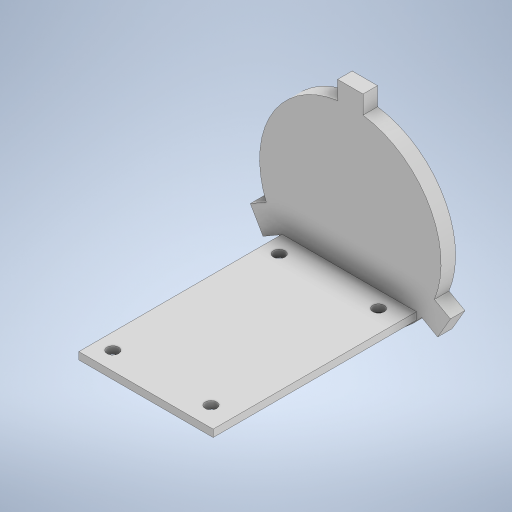
# Autodesk Inventor part: Electronic casing
Saved by Autodesk Inventor 2024 (Build 280153000, 153)
## iProperties
Created: 2024-03-27
Part Number: Electronic casing
Material: Generic
Document SubType Name: Modeling
Designer: auror
Density: 1 g/cm^3
Appearance: Default
Author: auror
Autodesk Inventor part; units mm, degrees
ref_plane "YZ Plane" through (0, 0, 0) normal (1, 0, 0) x (0, 1, 0)
ref_plane "XZ Plane" through (0, 0, 0) normal (0, 1, 0) x (-1, 0, 0)
ref_plane "XY Plane" through (0, 0, 0) normal (0, 0, 1) x (1, 0, 0)
sketch "Sketch2" plane through (0, 0, 0) normal (0, 1, 0) x (-1, 0, 0)
  line L0 (18.5, 28) -> (-18.5, 28)
  line L1 (-18.5, 28) -> (-18.5, -28)
  line L2 (-18.5, -28) -> (18.5, -28)
  line L3 (18.5, -28) -> (18.5, 28)
  point P0 (0, 0)
  point P1 (-18.5, 0)
  point P2 (18.5, 0)
  dimension "d0" = 37
  dimension "d1" = 56
  dimension "d2" = 28
  dimension "d3" = 18.5
  constraints: 8 end point, 2 midpoint, 2 parallel, 1 horizontal, 1 perpendicular
  measures "d0" distance of point (-18.5, 0) point (18.5, 0)
  measures "d1" distance between parallel lines of L2 L0
  measures "d2" distance from line of point (0, 0) L0
  measures "d3" distance from line of L3 point (0, 0)
extrude "Extrusion1" add sketch "Sketch2" along normal blind 2
sketch "Sketch3" plane through (0, 2, 0) normal (0, 1, 0) x (1, 0, 0)
  circle A0 centre (12.5, -22.6) radius 1.6
  circle A1 centre (-14.1006, -23.0348) radius 1.6
  circle A2 centre (-14.2118, 22.9033) radius 1.6
  circle A3 centre (12.5, 23.5707) radius 1.6
  point P0 (0, 0)
  dimension "d6" = 22.6
  dimension "d7" = 12.5
  dimension "d8" = 3.2
  dimension "d9" = 3.2
  dimension "d10" = 3.2
  dimension "d11" = 3.2
  constraints: 4 centre point, 4 coincident
  measures "d6" vertical distance of point (0, 0) point (12.5, -22.6)
  measures "d7" horizontal distance of point (0, 0) point (12.5, -22.6)
  measures "d8" diameter of A0
  measures "d9" diameter of A1
  measures "d10" diameter of A2
  measures "d11" diameter of A3
hole "Hole1" at (12.5, 2, 22.6) at (-14.1006, 2, 23.0348) at (-14.2118, 2, -22.9033) at (12.5, 2, -23.5707) direction (0, -1, 0) diameter 3.2 end through all
sketch "Sketch4" plane through (18.5, 0, -28) normal (0, 0, -1) x (-1, 0, 0)
  line L0 (0, 2.5) -> (37, 2.5) construction
  line L1 (18.2006, 41.8152) -> (18.2006, 0.4053) construction
  line L2 (18.2006, 16.8152) -> (-3.054, 4.5438) construction
  line L3 (18.2006, 16.8152) -> (18.2006, 41.8152) construction
  line L4 (18.2006, 16.8152) -> (39.8512, 4.3152) construction
  line L5 (14.7006, 46.6103) -> (14.7006, 41.569)
  line L6 (21.7006, 46.6103) -> (21.7006, 41.569)
  line L7 (14.7006, 46.6103) -> (21.7006, 46.6103)
  line L8 (-9.3679, 4.969) -> (-4.9773, 7.4458)
  line L9 (-5.8617, -1.0896) -> (-1.4711, 1.3872)
  line L10 (-9.3679, 4.969) -> (-5.8617, -1.0896)
  line L11 (41.3873, 7.4676) -> (45.7548, 4.9504)
  line L12 (37.8868, 1.4057) -> (42.2544, -1.1115)
  line L13 (42.2544, -1.1115) -> (45.7548, 4.9504)
  line L14 (18.2006, 16.8152) -> (-3.054, 4.5438) construction
  line L15 (27.389, 22.1201) -> (-3.054, 4.5438) construction
  line L16 (18.2006, 16.8152) -> (18.2006, 41.8152) construction
  line L17 (18.2006, 48.4448) -> (18.2006, 41.8152) construction
  line L18 (18.2006, 16.8152) -> (39.8512, 4.3152) construction
  line L19 (84.7852, -21.6275) -> (39.8512, 4.3152) construction
  arc A0 (-1.4711, 1.3872) -> (37.8868, 1.4057) centre (18.2006, 16.8152) ccw
  arc A1 (14.7006, 41.569) -> (-4.9773, 7.4458) centre (18.2006, 16.8152) ccw
  arc A2 (41.3873, 7.4676) -> (21.7006, 41.569) centre (18.2006, 16.8152) ccw
  line L20 (-0.2994, 0) -> (36.7006, 0) construction
  line L21 (0, 0) -> (37, 0) projected
  point P0 (18.5, 0)
  point P1 (-3.6664, 0.1488)
  point P2 (40.0706, 0.1471)
  point P3 (-7.1726, 6.2074)
  point P4 (21.7006, 44.0896)
  point P5 (43.571, 6.209)
  dimension "d32" = 7
  dimension "d33" = 7
  dimension "d34" = 7
  dimension "d37" = 3.5
  dimension "d38" = 3.5
  dimension "d39" = 3.5
  dimension "d40" = 5.0414
  dimension "d45" = 120
  dimension "d46" = 120
  dimension "d49" = 5.0414
  dimension "d51" = 5.041
  dimension "d52" = 5.041
  dimension "d53" = 5.041
  dimension "d54" = 5.041
  dimension "d55" = 7
  dimension "d56" = 7
  dimension "d57" = 7
  dimension "d58" = 25
  dimension "d59" = 25
  dimension "d60" = 25
  dimension "d61" = 37
  dimension "d62" = 0
  constraints: 42 end point, 17 point on circle, 5 collinear, 5 midpoint, 3 centre point, 3 point on line, 1 coincident, 1 horizontal, 1 vertical
  measures "d32" distance of point (-3.666, 0.149) point (-7.173, 6.207)
  measures "d33" distance from line of point (21.701, 44.09) L5
  measures "d34" distance of point (43.571, 6.209) point (40.071, 0.147)
  measures "d37" distance from line of L15 point (-3.666, 0.149)
  measures "d38" distance from line of point (21.701, 44.09) L17
  measures "d39" distance from line of L19 point (43.571, 6.209)
  measures "d40" distance of L5.start L5.end
  measures "d45" angle of L18 L3
  measures "d46" angle of L4 L15
  measures "d49" distance of L6.start L6.end
  measures "d51" distance of L8.start L8.end
  measures "d52" distance of L9.start L9.end
  measures "d53" distance of L11.end L11.start
  measures "d54" distance of L12.start L12.end
  measures "d55" distance of L9.end L8.end
  measures "d56" distance of L11.start L12.start
  measures "d57" distance of L6.end L5.end
  measures "d58" radius of A2
  measures "d59" radius of A0
  measures "d60" radius of A1
  measures "d61" distance of L20.start L20.end
  measures "d62" distance between parallel lines of L21 L20
extrude "Extrusion2" add sketch "Sketch4" along normal blind 4
body "Solid1"
